Autodesk Fusion 360 part; units mm, degrees
(part 2 of 2)
equation "d43 = -supp_wall_thickness / 2"
equation "d44 = supp_wall_thickness / 2"
equation "d45 = -supp_wall_thickness / 2"
equation "d46 = supp_wall_thickness / 2"
equation "d47 = -supp_wall_thickness / 2"
equation "d48 = supp_wall_thickness / 2"
equation "d49 = -supp_wall_thickness / 2"
equation "fence_fillet = 3 mm"
equation "plate2supp_screw_hole = 4 mm"
equation "d77 = fence_fillet"
equation "d78 = supp_wall_thickness"
equation "d79 = supp_wall_thickness"
equation "d80 = supp_wall_thickness"
equation "d81 = supp_wall_thickness"
equation "d85 = fence_fillet"
equation "d86 = supp_wall_thickness / 2"
equation "d87 = supp_wall_thickness / 2"
equation "d88 = supp_wall_thickness / 2"
equation "d89 = supp_wall_thickness / 2"
equation "d90 = supp_wall_thickness / 2"
equation "d91 = supp_wall_thickness / 2"
equation "d109 = base2supp_screw_outer"
equation "d110 = plate2supp_screw_hole"
equation "d114 = base2supp_screw_outer"
equation "d115 = plate2supp_screw_hole"
equation "d119 = plate2supp_screw_hole"
equation "d122 = plate2supp_screw_hole"
equation "d124 = wifi_screw_hole"
equation "d125 = wifi_screw_hole"
equation "wifi_screw_hole = 6.5 mm"
